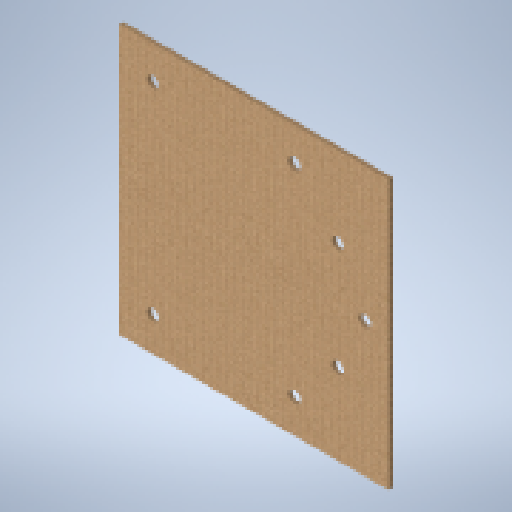
# Autodesk Inventor part: PortaTornillos
Saved by Autodesk Inventor 2023.1 (Build 271208000, 208)
## iProperties
Created: 2022-11-11
Part Number: PortaTornillos
Material: MDF Medium Density Fiberboard
Document SubType Name: Modeling
Designer: Daniel Peña
Density: 0.8 g/cm^3
Appearance: Cardboard - Corrugated
Author: Daniel Peña
Autodesk Inventor part; units mm, degrees
ref_plane "YZ Plane" through (0, 0, 0) normal (1, 0, 0) x (0, 1, 0)
ref_plane "XZ Plane" through (0, 0, 0) normal (0, 1, 0) x (-1, 0, 0)
ref_plane "XY Plane" through (0, 0, 0) normal (0, 0, 1) x (1, 0, 0)
sketch "Sketch1" plane through (0, 0, 0) normal (0, 0, 1) x (1, 0, 0)
  line L0 (-100, -100) -> (100, -100) projected
  line L1 (100, -100) -> (100, 100) projected
  line L2 (100, 100) -> (-100, 100) projected
  line L3 (-100, 100) -> (-100, -100) projected
  point P0 (0, 0)
extrude "Extrusion1" add sketch "Sketch1" along normal blind 3
sketch "Sketch2" plane through (0, 0, 3) normal (0, 0, 1) x (1, 0, 0)
  point P0 (0, 0)
  point P1 (-75, 75)
  point P2 (30, 75)
  point P3 (62.5, 40)
  point P4 (82.5001, 0)
  point P5 (62.5, -40)
  point P6 (30, -75)
  point P7 (-75, -75)
hole "Hole1" at (-75, 75, 3) at (30, 75, 3) at (62.5, 40, 3) at (82.5001, 0, 3) at (62.5, -40, 3) at (30, -75, 3) at (-75, -75, 3) direction (0, 0, -1) diameter 8.3 end through all
body "Solid1"
